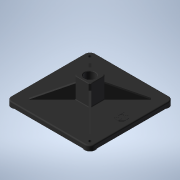
# Autodesk Inventor part: BZB-FP
Saved by Autodesk Inventor 2021 (Build 250183000, 183)
## iProperties
Created: 2025-06-23
Part Number: BZB-FP
Material: Generic
Catalog Web Link: www.cadenas.de
Description: base stand BZB-Accessories
Vendor: RNA
Document SubType Name: Modeling
Designer: psAdmin
Manufacturer: RNA
Mass: 4034.2 g
Surface Area: 4370.34 cm^2
Volume: 4034.2 cm^3
Density: 1 g/cm^3
Appearance: PSOLRGB-175-175-175
Category: PARTsolutions
Company: RNA
Title: BZB-FP
Author: Cadenas PARTsolutions
Comments: Accessories
PSOL_IDENT_0: {$CADENAS_DATA/23d-libs/rna/bunker/zubehoer/parts/bzb_fussplatte.prj},160 {VTYP=3D},{NB=BZB-FP},{LIN
PSOL_IDENT_1: A=BZB-FP},{NN=base stand BZB},{DATE=06.06.2017 07:14:33},{GEOMDATE=23.02.2017 07:08:00},{VERSION=},{
PSOL_IDENT_2: LINEID=10},{WBVAR=},{WBNUMERIC=}  {NB=BZB-FP},{LINA=BZB-FP},{KT=DUMMY},{IDNR=BZB-FP}
NB: BZB-FP
NN: base stand BZB
NT: Accessories
NBSYN: $IDNR.
LINA: BZB-FP
CATALOG: Rhein-Nadel-Automation
IDNR: BZB-FP
SUPPLIER: RNA
ARTICLENO: BZB-FP
BOMINFO: BZB-FP
CREATOR: CADENAS GmbH
Autodesk Inventor part; units mm, degrees
sketch "Sketch_1" plane through (0, 0, 0) normal (0, 0, 1) x (1, 0, 0)
  line L0 (-200, 20) -> (-200, 3)
  line L1 (-200, 3) -> (200, 3)
  line L2 (200, 3) -> (200, 20)
  arc A0 (200, 20) -> (195, 25) centre (195, 20) ccw
  line L3 (195, 25) -> (-195, 25)
  arc A1 (-195, 25) -> (-200, 20) centre (-195, 20) ccw
  constraints: 8 end point, 4 point on circle, 2 centre point
extrude "Extrusion1" add sketch "Sketch_1" along normal mid plane 350
sketch "Sketch_2" plane through (0, 0, 0) normal (1, 0, 0) x (0, 1, 0)
  line L0 (20, 200) -> (3, 200)
  line L1 (3, 200) -> (3, -200)
  line L2 (3, -200) -> (20, -200)
  arc A0 (20, -200) -> (25, -195) centre (20, -195) ccw
  line L3 (25, -195) -> (25, 195)
  arc A1 (25, 195) -> (20, 200) centre (20, 195) ccw
  constraints: 8 end point, 4 point on circle, 2 centre point
extrude "Extrusion2" add sketch "Sketch_2" along normal mid plane 350
sketch "Sketch_3" plane through (0, 0, 175) normal (0, 0, 1) x (1, 0, 0)
  line L0 (175, 3) -> (175, 25)
  line L1 (175, 25) -> (195, 25)
  arc A0 (200, 20) -> (195, 25) centre (195, 20) ccw
  line L2 (200, 20) -> (200, 3)
  line L3 (200, 3) -> (175, 3)
  line L4 (175, 3) -> (175, 25)
  constraints: 10 end point, 2 point on circle, 1 centre point
revolve "Revolution1" add sketch "Sketch_3" angle 90 about axis through (175, 3, 175) along (0, -1, 0)
sketch "Sketch_4" plane through (0, 0, 175) normal (0, 0, 1) x (1, 0, 0)
  line L0 (-175, 25) -> (-175, 3)
  line L1 (-175, 3) -> (-200, 3)
  line L2 (-200, 3) -> (-200, 20)
  arc A0 (-195, 25) -> (-200, 20) centre (-195, 20) ccw
  line L3 (-195, 25) -> (-175, 25)
  line L4 (-175, 25) -> (-175, 3)
  constraints: 10 end point, 2 point on circle, 1 centre point
revolve "Revolution2" add sketch "Sketch_4" angle 90 about axis through (-175, 25, 175) along (0, 1, 0)
sketch "Sketch_5" plane through (0, 0, -175) normal (0, 0, 1) x (1, 0, 0)
  line L0 (175, 3) -> (175, 25)
  line L1 (175, 25) -> (195, 25)
  arc A0 (200, 20) -> (195, 25) centre (195, 20) ccw
  line L2 (200, 20) -> (200, 3)
  line L3 (200, 3) -> (175, 3)
  line L4 (175, 3) -> (175, 25)
  constraints: 10 end point, 2 point on circle, 1 centre point
revolve "Revolution3" add sketch "Sketch_5" angle 90 about axis through (175, 3, -175) along (0, 1, 0)
sketch "Sketch_6" plane through (0, 0, -175) normal (0, 0, 1) x (1, 0, 0)
  line L0 (-175, 25) -> (-175, 3)
  line L1 (-175, 3) -> (-200, 3)
  line L2 (-200, 3) -> (-200, 20)
  arc A0 (-195, 25) -> (-200, 20) centre (-195, 20) ccw
  line L3 (-195, 25) -> (-175, 25)
  line L4 (-175, 25) -> (-175, 3)
  constraints: 10 end point, 2 point on circle, 1 centre point
revolve "Revolution4" add sketch "Sketch_6" angle 90 about axis through (-175, 25, -175) along (0, -1, 0)
sketch "Sketch_7" plane through (0, 0, 175) normal (0, 0, 1) x (1, 0, 0)
  line L0 (175, 0) -> (175, 3)
  line L1 (175, 3) -> (203, 3)
  arc A0 (203, 3) -> (200, 0) centre (203, 0) ccw
  line L2 (200, 0) -> (175, 0)
  line L3 (175, 0) -> (175, 3)
  constraints: 8 end point, 2 point on circle, 1 centre point
revolve "Revolution5" add sketch "Sketch_7" angle 360 about axis through (175, 0, 175) along (0, -1, 0)
sketch "Sketch_8" plane through (0, 0, 175) normal (0, 0, 1) x (1, 0, 0)
  line L0 (-175, 0) -> (-175, 3)
  line L1 (-175, 3) -> (-147, 3)
  arc A0 (-147, 3) -> (-150, 0) centre (-147, 0) ccw
  line L2 (-150, 0) -> (-175, 0)
  line L3 (-175, 0) -> (-175, 3)
  constraints: 8 end point, 2 point on circle, 1 centre point
revolve "Revolution6" add sketch "Sketch_8" angle 360 about axis through (-175, 0, 175) along (0, -1, 0)
sketch "Sketch_9" plane through (0, 0, -175) normal (0, 0, 1) x (1, 0, 0)
  line L0 (175, 0) -> (175, 3)
  line L1 (175, 3) -> (203, 3)
  arc A0 (203, 3) -> (200, 0) centre (203, 0) ccw
  line L2 (200, 0) -> (175, 0)
  line L3 (175, 0) -> (175, 3)
  constraints: 8 end point, 2 point on circle, 1 centre point
revolve "Revolution7" add sketch "Sketch_9" angle 360 about axis through (175, 0, -175) along (0, -1, 0)
sketch "Sketch_10" plane through (0, 0, -175) normal (0, 0, 1) x (1, 0, 0)
  line L0 (-175, 0) -> (-175, 3)
  line L1 (-175, 3) -> (-147, 3)
  arc A0 (-147, 3) -> (-150, 0) centre (-147, 0) ccw
  line L2 (-150, 0) -> (-175, 0)
  line L3 (-175, 0) -> (-175, 3)
  constraints: 8 end point, 2 point on circle, 1 centre point
revolve "Revolution8" add sketch "Sketch_10" angle 360 about axis through (-175, 0, -175) along (0, -1, 0)
sketch "Sketch_12" plane through (0, 3, 0) normal (0, 1, 0) x (1, 0, 0)
  line L0 (-300, -300) -> (300, -300)
  line L1 (300, -300) -> (300, 300)
  line L2 (300, 300) -> (-300, 300)
  line L3 (-300, 300) -> (-300, -300)
  arc A0 (-200, -175) -> (-175, -200) centre (-175, -175) ccw
  line L4 (-175, -200) -> (175, -200)
  arc A1 (175, -200) -> (200, -175) centre (175, -175) ccw
  line L5 (200, -175) -> (200, 175)
  arc A2 (200, 175) -> (175, 200) centre (175, 175) ccw
  line L6 (175, 200) -> (-175, 200)
  arc A3 (-175, 200) -> (-200, 175) centre (-175, 175) ccw
  line L7 (-200, 175) -> (-200, -175)
  constraints: 16 end point, 8 point on circle, 4 centre point
extrude "Extrusion3" cut sketch "Sketch_12" along normal mid plane 100
sketch "Sketch12" plane through (-175, 0, -175) normal (0, -1, 0) x (0.7071, 0, 0.7071)
  point P0 (0, 0)
hole "Hole1" at (-175, 0, -175) direction (0, 1, 0) diameter 13 depth 50
sketch "Sketch13" plane through (175, 0, 175) normal (0, -1, 0) x (0.7071, 0, 0.7071)
  point P0 (0, 0)
hole "Hole2" at (175, 0, 175) direction (0, 1, 0) diameter 13 depth 50
sketch "Sketch_14" plane through (0, 0, 0) normal (0.7071, 0, 0.7071) x (0.7071, 0, -0.7071)
  line L0 (-205.8751, 25) -> (205.8751, 25)
  line L1 (205.8751, 25) -> (0, 112.3888)
  line L2 (0, 112.3888) -> (-205.8751, 25)
  constraints: 6 end point
extrude "Extrusion4" add sketch "Sketch_14" along normal mid plane 10
sketch "Sketch_15" plane through (0, 0, 0) normal (0.7071, 0, -0.7071) x (-0.7071, 0, -0.7071)
  line L0 (-205.8751, 25) -> (205.8751, 25)
  line L1 (205.8751, 25) -> (0, 112.3888)
  line L2 (0, 112.3888) -> (-205.8751, 25)
  constraints: 6 end point
extrude "Extrusion5" add sketch "Sketch_15" along normal mid plane 10
sketch "Sketch_16" plane through (0, 25, 0) normal (0, 1, 0) x (1, 0, 0)
  line L0 (-37.5, -30.4289) -> (-30.4289, -37.5)
  line L1 (-30.4289, -37.5) -> (30.4289, -37.5)
  line L2 (30.4289, -37.5) -> (37.5, -30.4289)
  line L3 (37.5, -30.4289) -> (37.5, 30.4289)
  line L4 (37.5, 30.4289) -> (30.4289, 37.5)
  line L5 (30.4289, 37.5) -> (-30.4289, 37.5)
  line L6 (-30.4289, 37.5) -> (-37.5, 30.4289)
  line L7 (-37.5, 30.4289) -> (-37.5, -30.4289)
  constraints: 16 end point
extrude "Extrusion6" add sketch "Sketch_16" along normal blind 97
sketch "Sketch_24" plane through (0, 0, 0) normal (0, 0, 1) x (1, 0, 0)
  line L0 (-40.5, 25) -> (40.5, 25)
  arc A0 (37.5, 28) -> (40.5, 25) centre (40.5, 28) ccw
  line L1 (37.5, 28) -> (-37.5, 28)
  arc A1 (-40.5, 25) -> (-37.5, 28) centre (-40.5, 28) ccw
  constraints: 4 end point, 4 point on circle, 2 centre point
extrude "Extrusion7" add sketch "Sketch_24" along normal mid plane 75
sketch "Sketch_25" plane through (0, 0, 0) normal (1, 0, 0) x (0, 1, 0)
  line L0 (25, 40.5) -> (25, -40.5)
  arc A0 (28, -37.5) -> (25, -40.5) centre (28, -40.5) ccw
  line L1 (28, -37.5) -> (28, 37.5)
  arc A1 (25, 40.5) -> (28, 37.5) centre (28, 40.5) ccw
  constraints: 4 end point, 4 point on circle, 2 centre point
extrude "Extrusion8" add sketch "Sketch_25" along normal mid plane 75
sketch "Sketch_17" plane through (0, 0, 0) normal (0.7071, 0, 0.7071) x (0.7071, 0, -0.7071)
  line L0 (-53.033, 120) -> (-48.033, 120)
  line L1 (-48.033, 120) -> (-46.033, 122)
  line L2 (-46.033, 122) -> (46.033, 122)
  line L3 (46.033, 122) -> (48.033, 120)
  line L4 (48.033, 120) -> (53.033, 120)
  line L5 (53.033, 120) -> (53.033, 127)
  line L6 (53.033, 127) -> (-53.033, 127)
  line L7 (-53.033, 127) -> (-53.033, 120)
  constraints: 16 end point
sketch "Sketch_18" plane through (0, 0, 0) normal (0.7071, 0, -0.7071) x (-0.7071, 0, -0.7071)
  line L0 (-53.033, 120) -> (-48.033, 120)
  line L1 (-48.033, 120) -> (-46.033, 122)
  line L2 (-46.033, 122) -> (46.033, 122)
  line L3 (46.033, 122) -> (48.033, 120)
  line L4 (48.033, 120) -> (53.033, 120)
  line L5 (53.033, 120) -> (53.033, 127)
  line L6 (53.033, 127) -> (-53.033, 127)
  line L7 (-53.033, 127) -> (-53.033, 120)
  constraints: 16 end point
sketch "Sketch_19" plane through (0, 0, 0) normal (0, 0, 1) x (1, 0, 0)
  line L0 (-42.5, 127) -> (-42.5, 117)
  line L1 (-42.5, 117) -> (-37.5, 117)
  line L2 (-37.5, 117) -> (-37.5, 120)
  line L3 (-37.5, 120) -> (-35.5, 122)
  line L4 (-35.5, 122) -> (35.5, 122)
  line L5 (35.5, 122) -> (37.5, 120)
  line L6 (37.5, 120) -> (37.5, 117)
  line L7 (37.5, 117) -> (42.5, 117)
  line L8 (42.5, 117) -> (42.5, 127)
  line L9 (42.5, 127) -> (-42.5, 127)
  constraints: 20 end point
extrude "Extrusion9" cut sketch "Sketch_19" along normal mid plane 80
sketch "Sketch_20" plane through (0, 0, 0) normal (1, 0, 0) x (0, 1, 0)
  line L0 (127, 42.5) -> (117, 42.5)
  line L1 (117, 42.5) -> (117, 37.5)
  line L2 (117, 37.5) -> (120, 37.5)
  line L3 (120, 37.5) -> (122, 35.5)
  line L4 (122, 35.5) -> (122, -35.5)
  line L5 (122, -35.5) -> (120, -37.5)
  line L6 (120, -37.5) -> (117, -37.5)
  line L7 (117, -37.5) -> (117, -42.5)
  line L8 (117, -42.5) -> (127, -42.5)
  line L9 (127, -42.5) -> (127, 42.5)
  constraints: 20 end point
extrude "Extrusion10" cut sketch "Sketch_20" along normal mid plane 80
sketch "Sketch23" plane through (0, 122, 0) normal (0, 1, 0) x (1, 0, 0)
  point P0 (0, 0)
hole "Hole3" at (0, 122, 0) direction (0, -1, 0) diameter 50 depth 117 countersink diameter 54 countersink angle 90
sketch "Sketch_22" plane through (0, 0, 0) normal (0.7071, 0, -0.7071) x (-0.7071, 0, -0.7071)
  circle A0 centre (0, 110) radius 4.25
  constraints: 1 centre point
extrude "Extrusion11" cut sketch "Sketch_22" along normal blind 100
sketch "Sketch_23" plane through (0, 0, 0) normal (0, 1, 0) x (-1, 0, 0)
  line L0 (17.6777, 17.6777) -> (-17.6777, 17.6777)
  line L1 (-17.6777, 17.6777) -> (-17.6777, -17.6777)
  line L2 (-17.6777, -17.6777) -> (17.6777, -17.6777)
  line L3 (17.6777, -17.6777) -> (17.6777, 17.6777)
  constraints: 8 end point
extrude "Extrusion12" cut sketch "Sketch_23" along normal blind 5
extrude "Extrusion13" cut sketch "Sketch_17" along normal mid plane 30
extrude "Extrusion14" cut sketch "Sketch_18" along normal mid plane 30
sketch "Sketch_29" plane through (0, 25, 0) normal (0, 1, 0) x (1, 0, 0)
  line L0 (161.2, -24.855) -> (174.77, -11.285)
  line L1 (174.77, -11.285) -> (174.77, -3.755)
  line L2 (174.77, -3.755) -> (161.2, 4.0796)
  line L3 (161.2, 4.0796) -> (161.2, -24.855)
  constraints: 8 end point
extrude "Extrusion15" add sketch "Sketch_29" along normal blind 2
sketch "Sketch_30" plane through (0, 25, 0) normal (0, 1, 0) x (1, 0, 0)
  line L0 (150.517, 11.7948) -> (174.77, -2.2077)
  line L1 (174.77, -2.2077) -> (174.77, 10.355)
  line L2 (174.77, 10.355) -> (164.98, 20.145)
  line L3 (164.98, 20.145) -> (150.517, 11.7948)
  constraints: 8 end point
extrude "Extrusion16" add sketch "Sketch_30" along normal blind 2
sketch "Sketch_31" plane through (0, 25, 0) normal (0, 1, 0) x (1, 0, 0)
  line L0 (135.8016, -21.0566) -> (139.6, -24.855)
  line L1 (139.6, -24.855) -> (159.88, -24.855)
  line L2 (159.88, -24.855) -> (159.88, -7.155)
  line L3 (159.88, -7.155) -> (135.8016, -21.0566)
  constraints: 8 end point
extrude "Extrusion17" add sketch "Sketch_31" along normal blind 2
sketch "Sketch_32" plane through (0, 25, 0) normal (0, 1, 0) x (1, 0, 0)
  line L0 (125.1, 2.2077) -> (125.1, -10.355)
  line L1 (125.1, -10.355) -> (134.89, -20.145)
  line L2 (134.89, -20.145) -> (149.353, -11.7948)
  line L3 (149.353, -11.7948) -> (125.1, 2.2077)
  constraints: 8 end point
extrude "Extrusion18" add sketch "Sketch_32" along normal blind 2
sketch "Sketch_33" plane through (0, 25, 0) normal (0, 1, 0) x (1, 0, 0)
  line L0 (125.1, 11.285) -> (125.1, 3.755)
  line L1 (125.1, 3.755) -> (138.67, -4.0796)
  line L2 (138.67, -4.0796) -> (138.67, 24.855)
  line L3 (138.67, 24.855) -> (125.1, 11.285)
  constraints: 8 end point
extrude "Extrusion19" add sketch "Sketch_33" along normal blind 2
sketch "Sketch_34" plane through (0, 25, 0) normal (0, 1, 0) x (1, 0, 0)
  line L0 (139.99, 7.155) -> (164.0684, 21.0566)
  line L1 (164.0684, 21.0566) -> (160.27, 24.855)
  line L2 (160.27, 24.855) -> (139.99, 24.855)
  line L3 (139.99, 24.855) -> (139.99, 7.155)
  constraints: 8 end point
extrude "Extrusion20" add sketch "Sketch_34" along normal blind 2
ref_plane "DUMMY_XY" through (0, 0, 0) normal (0, 1, 0) x (1, 0, 0)
ref_plane "DUMMY_YZ" through (0, 0, 0) normal (1, 0, 0) x (0, 0, -1)
ref_plane "DUMMY_ZX" through (0, 0, 0) normal (0, 0, -1) x (0, 1, 0)
ref_plane "PROFIL_XY" through (0, 5, 0) normal (0, -1, 0) x (1, 0, 0)
ref_plane "PROFIL_YZ" through (0, 5, 0) normal (1, 0, 0) x (0, 0, 1)
ref_plane "PROFIL_ZX" through (0, 5, 0) normal (0, 0, 1) x (0, -1, 0)
ref_plane "PROFIL2_XY" through (0, 122, 0) normal (0, -1, 0) x (1, 0, 0)
ref_plane "PROFIL2_YZ" through (0, 122, 0) normal (1, 0, 0) x (0, 0, 1)
ref_plane "PROFIL2_ZX" through (0, 122, 0) normal (0, 0, 1) x (0, -1, 0)
body "Solid1"
